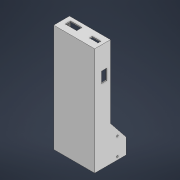
# Autodesk Inventor part: uHousing
Saved by Autodesk Inventor 2021 (Build 250183000, 183)
## iProperties
Created: 2023-04-08
Part Number: uHousing
Material: Generic
Document SubType Name: Modeling
Designer: ivanl
Density: 1 g/cm^3
Appearance: Default
Author: ivanl
## iProperties of the stored document _3DPrint.ipt
Created: 2023-04-08
Part Number: _3DPrint
Material: Generic
Document SubType Name: Modeling
Designer: ivanl
Density: 1 g/cm^3
Appearance: Default
Author: ivanl
Autodesk Inventor part; units mm, degrees
ref_plane "YZ Plane" through (0, 0, 0) normal (1, 0, 0) x (0, 1, 0)
ref_plane "XZ Plane" through (0, 0, 0) normal (0, 1, 0) x (-1, 0, 0)
ref_plane "XY Plane" through (0, 0, 0) normal (0, 0, 1) x (1, 0, 0)
sketch "Sketch1" plane through (0, 0, 0) normal (0, 0, 1) x (1, 0, 0)
  line L0 (0, 0) -> (64.77, 0)
  line L1 (64.77, 0) -> (64.77, 175.26)
  line L2 (64.77, 175.26) -> (0, 175.26)
  line L3 (0, 175.26) -> (0, 0)
  dimension "d0" = 64.77
  dimension "d1" = 175.26
  constraints: 8 end point, 2 parallel, 1 horizontal, 1 perpendicular
  measures "d0" distance of L0.start L0.end
  measures "d1" distance of L0.end L1.end
extrude "Extrusion1" add sketch "Sketch1" along normal blind 50.8
shell "Shell1" thickness 1.5875 outward yes removed faces 1 at (21.59, 116.84, 0)
sketch "Sketch2" plane through (0, 175.26, 0) normal (0, -1, 0) x (1, 0, 0)
  line L0 (64.77, 50.8) -> (0, 50.8) projected
  line L1 (64.77, 50.8) -> (0, 50.8)
  line L2 (0, 50.8) -> (0, 41.275)
  line L3 (0, 41.275) -> (64.77, 41.275)
  line L4 (64.77, 41.275) -> (64.77, 50.8)
  line L5 (60.706, 41.275) -> (46.482, 41.275)
  line L6 (46.482, 41.275) -> (46.482, 36.5125)
  line L7 (46.482, 36.5125) -> (60.706, 36.5125)
  line L8 (60.706, 36.5125) -> (60.706, 41.275)
  line L9 (25.4, 41.275) -> (6.35, 41.275)
  line L10 (6.35, 41.275) -> (6.35, 32.385)
  line L11 (6.35, 32.385) -> (25.4, 32.385)
  line L12 (25.4, 32.385) -> (25.4, 41.275)
  point P0 (0, 0)
  point P1 (6.35, 41.275)
  dimension "d5" = 9.525
  dimension "d6" = 64.77
  dimension "d7" = 4.7625
  dimension "d8" = 14.224
  dimension "d9" = 18.288
  dimension "d10" = 19.05
  dimension "d11" = 25.4
  dimension "d12" = 8.89
  constraints: 24 end point, 6 parallel, 3 horizontal, 3 perpendicular, 2 point on line
  measures "d5" distance of L2.end L1.end
  measures "d6" distance of L2.end L3.end
  measures "d7" distance of L6.end L5.end
  measures "d8" distance of L6.end L7.end
  measures "d9" distance between parallel lines of L4 L6
  measures "d10" distance of L11.end L10.end
  measures "d11" distance between parallel lines of L2 L12
  measures "d12" distance of L11.end L9.start
sketch "Sketch4" plane through (0, 0, 0) normal (0, 1, 0) x (1, 0, 0)
  line L0 (0, 0) -> (0, -50.8) projected
  line L1 (0, -50.8) -> (64.77, -50.8)
  line L2 (64.77, -50.8) -> (64.77, -41.275)
  line L3 (64.77, -41.275) -> (0, -41.275)
  line L4 (0, -41.275) -> (0, -50.8)
  line L5 (37.7825, -41.275) -> (60.0075, -41.275)
  line L6 (60.0075, -41.275) -> (60.0075, -25.4)
  line L7 (60.0075, -25.4) -> (37.7825, -25.4)
  line L8 (37.7825, -25.4) -> (37.7825, -41.275)
  line L9 (20.6375, -41.275) -> (33.3375, -41.275)
  line L10 (33.3375, -41.275) -> (33.3375, -34.925)
  line L11 (33.3375, -34.925) -> (20.6375, -34.925)
  line L12 (20.6375, -34.925) -> (20.6375, -41.275)
  dimension "d13" = 9.525
  dimension "d14" = 64.77
  dimension "d15" = 22.225
  dimension "d16" = 15.875
  dimension "d17" = 26.9875
  dimension "d18" = 12.7
  dimension "d19" = 6.35
  dimension "d20" = 33.3375
  constraints: 24 end point, 6 parallel, 3 horizontal, 3 perpendicular, 2 point on line
  measures "d13" distance of L2.end L1.end
  measures "d14" distance of L2.end L3.end
  measures "d15" distance of L7.end L6.end
  measures "d16" distance of L7.end L5.start
  measures "d17" distance between parallel lines of L2 L8
  measures "d18" distance of L10.end L11.end
  measures "d19" distance of L11.end L9.start
  measures "d20" distance between parallel lines of L0 L10
sketch "Sketch5" plane through (0, 0, 0) normal (1, 0, 0) x (0, 0, -1)
  line L0 (-50.8, 175.26) -> (-50.8, 0) projected
  line L1 (-50.8, 175.26) -> (-41.275, 175.26)
  line L2 (-41.275, 175.26) -> (-41.275, 0)
  line L3 (-41.275, 0) -> (-50.8, 0)
  line L4 (-50.8, 0) -> (-50.8, 175.26)
  line L5 (-41.275, 139.192) -> (-32.385, 139.192)
  line L6 (-32.385, 139.192) -> (-32.385, 121.412)
  line L7 (-32.385, 121.412) -> (-41.275, 121.412)
  line L8 (-41.275, 121.412) -> (-41.275, 139.192)
  point P0 (0, 0)
  dimension "d21" = 9.525
  dimension "d22" = 175.26
  dimension "d23" = 17.78
  dimension "d24" = 8.89
  dimension "d25" = 53.848
  constraints: 16 end point, 4 parallel, 2 horizontal, 2 perpendicular, 1 point on line
  measures "d21" distance of L2.end L3.end
  measures "d22" distance of L1.end L2.end
  measures "d23" distance of L5.end L6.end
  measures "d24" distance of L6.end L7.end
  measures "d25" distance between parallel lines of L1 L7
extrude "Extrusion2" cut sketch "Sketch5" along normal mid plane 171.45 contours L5 L6 L7 L2
extrude "Extrusion3" cut sketch "Sketch2" against normal blind 171.45 contours L8 L7 L6 L3 | L3 L12 L11 L10
extrude "Extrusion4" cut sketch "Sketch4" against normal blind 171.45 contours L12 L11 L10 L3 | L8 L7 L6 L3
sketch "Sketch6" plane through (-1.5875, -1.5875, 0) normal (-1, 0, 0) x (0, 0, 1)
  line L0 (0, 0) -> (52.3875, 0) projected
  line L1 (0, 0) -> (0, 25.4)
  line L2 (0, 176.8475) -> (0, 1.5875) projected
  line L3 (0, 25.4) -> (26.1938, 58.1347)
  line L4 (26.1938, 58.1347) -> (26.1938, 178.435)
  line L5 (0, 178.435) -> (52.3875, 178.435) projected
  line L6 (0, 178.435) -> (0, 25.4)
  dimension "d32" = 25.4
  constraints: 8 end point, 1 midpoint, 1 point on line
  measures "d32" distance of L0.start L1.end
extrude "Extrusion5" cut sketch "Sketch6" against normal blind 171.45
sketch "Sketch7" plane through (-1.5875, -1.5875, 0) normal (0, -1, 0) x (1, 0, 0)
  circle A0 centre (5.207, 18.4912) radius 2.25
  line L0 (0, 0) -> (0, 52.3875) projected
  line L1 (0, 0) -> (67.945, 0) projected
  circle A1 centre (40.207, 18.4912) radius 2.25
  point P0 (1.5875, 0)
  dimension "d35" = 4.5
  dimension "d36" = 5.207
  dimension "d37" = 18.4912
  dimension "d38" = 4.5
  dimension "d39" = 35
  constraints: 2 centre point
  measures "d35" diameter of A0
  measures "d36" distance from line of L0 A0.centre
  measures "d37" distance from line of L1 A0.centre
  measures "d38" diameter of A1
  measures "d39" distance of A0.centre A1.centre
extrude "Extrusion6" cut sketch "Sketch7" against normal blind 171.45
sketch "Sketch8" plane through (-1.5875, -1.5875, 0) normal (0, -1, 0) x (1, 0, 0)
  circle A0 centre (22.707, 26.4912) radius 5.5
  circle A1 centre (5.207, 18.4912) radius 2.25 projected
  point P0 (1.5875, 0)
  dimension "d42" = 11
  dimension "d43" = 8
  dimension "d44" = 17.5
  constraints: 1 centre point
  measures "d42" diameter of A0
  measures "d43" vertical distance of A1.centre A0.centre
  measures "d44" horizontal distance of A1.centre A0.centre
extrude "Extrusion7" cut sketch "Sketch8" against normal blind 10 contours A0
sketch "Sketch9" plane through (66.3575, -1.5875, 52.3875) normal (1, 0, 0) x (0, 0, -1)
  circle A0 centre (37.3875, 5) radius 1.5
  circle A1 centre (37.3875, 34.5) radius 1.5
  line L0 (52.3875, 0) -> (0, 0) projected
  line L1 (52.3875, 0) -> (52.3875, 25.4) projected
  point P0 (52.3875, 1.5875)
  dimension "d47" = 3
  dimension "d48" = 3
  dimension "d49" = 29.5
  dimension "d50" = 5
  dimension "d51" = 15
  dimension "d52" = 15
  constraints: 2 centre point
  measures "d47" diameter of A0
  measures "d48" diameter of A1
  measures "d49" distance of A0.centre A1.centre
  measures "d50" distance from line of L0 A0.centre
  measures "d51" distance from line of L1 A0.centre
  measures "d52" distance from line of L1 A1.centre
extrude "Extrusion8" cut sketch "Sketch9" against normal blind 10
body "Solid1"
